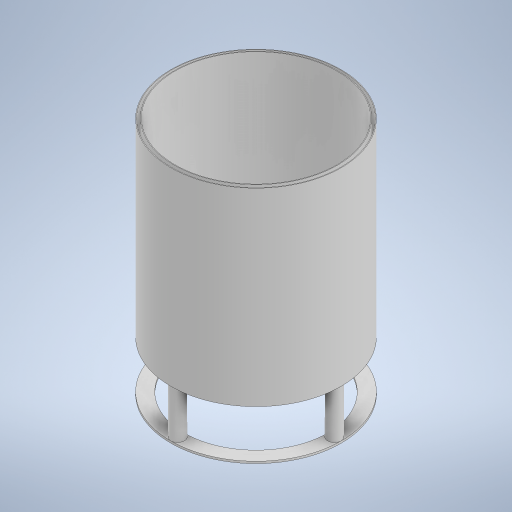
# Autodesk Inventor part: Mäskmaskin
Saved by Autodesk Inventor 2024 (Build 280153000, 153)
## iProperties
Created: 2024-02-28
Part Number: Mäskmaskin
Material: Generic
Document SubType Name: Modeling
Designer: Emil
Density: 1 g/cm^3
Appearance: Default
Mass: 881.668 g
Surface Area: 10423.6 cm^2
Volume: 881.668 cm^3
Author: Emil
Autodesk Inventor part; units mm, degrees
ref_plane "YZ Plane" through (0, 0, 0) normal (1, 0, 0) x (0, 1, 0)
ref_plane "XZ Plane" through (0, 0, 0) normal (0, 1, 0) x (-1, 0, 0)
ref_plane "XY Plane" through (0, 0, 0) normal (0, 0, 1) x (1, 0, 0)
sketch "Sketch1" plane through (0, 0, 0) normal (0, 1, 0) x (-1, 0, 0)
  circle A0 centre (0, 0) radius 125
  circle A1 centre (0, 0) radius 126
  dimension "d0" = 250
  dimension "d1" = 252
  constraints: 2 centre point, 2 coincident
  measures "d0" diameter of A0
  measures "d1" diameter of A1
extrude "Extrusion1" add sketch "Sketch1" along normal mid plane 280
sketch "Sketch3" plane through (0, -140, 0) normal (0, -1, 0) x (1, 0, 0)
  circle A0 centre (0, 0) radius 126
  dimension "d32" = 252
  constraints: 1 centre point, 1 coincident
  measures "d32" diameter of A0
extrude "Extrusion3" add sketch "Sketch3" against normal blind 1
sketch "Sketch8" plane through (0, -140, 0) normal (0, -1, 0) x (1, 0, 0)
  circle A0 centre (0, 0) radius 60
  circle A1 centre (0, 0) radius 59
  dimension "d18" = 120
  dimension "d43" = 118
  constraints: 2 centre point, 2 coincident
  measures "d18" diameter of A0
  measures "d43" diameter of A1
extrude "Extrusion8" add sketch "Sketch8" along normal blind 30
sketch "Sketch9" plane through (0, -140, 0) normal (0, -1, 0) x (1, 0, 0)
  point P0 (0, 0)
sketch "Sketch10" plane through (0, -140, 0) normal (0, -1, 0) x (1, 0, 0)
  circle A0 centre (116, 0) radius 10
  circle A1 centre (0, 0) radius 126 projected
  circle A2 centre (116, 0) radius 9
  dimension "d35" = 20
  dimension "d42" = 18
  constraints: 2 centre point, 1 coincident, 1 tangent
  measures "d35" diameter of A0
  measures "d42" diameter of A2
extrude "Extrusion9" add sketch "Sketch10" along normal blind 70 contours A0
pattern_circular "Circular Pattern1" count 4 over 360 about axis through (0, -10, 0) along (0, 1, 0) of "Extrusion9", "Extrusion3"
sketch "Sketch12" plane through (0, -139, 0) normal (0, 1, 0) x (1, 0, 0)
  circle A0 centre (0, 0) radius 120
  circle A1 centre (0, 0) radius 121
  dimension "d28" = 240
  dimension "d29" = 242
  constraints: 2 centre point, 2 coincident
  measures "d28" diameter of A0
  measures "d29" diameter of A1
extrude "Extrusion12" add sketch "Sketch12" along normal blind 280
sketch "Sketch13" plane through (0, -210, 116) normal (0, -1, 0) x (1, 0, 0)
  circle A0 centre (0, -116) radius 106
  circle A1 centre (0, -116) radius 126.0249
  point P0 (0, 10)
  dimension "d38" = 212
  dimension "d39" = 252.0497
  constraints: 2 centre point, 2 coincident
  measures "d38" diameter of A0
  measures "d39" diameter of A1
extrude "Extrusion14" add sketch "Sketch13" along normal blind 3
sketch "Sketch14" plane through (0, -170, 0) normal (0, -1, 0) x (1, 0, 0)
  circle A0 centre (0, 0) radius 60
  constraints: 1 centre point, 1 coincident
extrude "Extrusion15" add sketch "Sketch14" along normal blind 1
body "Solid1"
